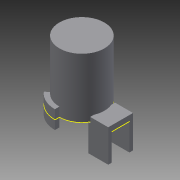
# Autodesk Inventor part: 知能ロボコンシリンダ延長
Saved by Autodesk Inventor 2013 (Build 170138000, 138)
## iProperties
Created: 2014-06-19
Part Number: 知能ロボコンシリンダ延長
Material: 一般
Document SubType Name: Modeling
Designer: horumo136
Density: 1 g/cm^3
Author: horumo136
Autodesk Inventor part; units mm, degrees
ref_plane "YZ Plane" through (0, 0, 0) normal (1, 0, 0) x (0, 1, 0)
ref_plane "XZ Plane" through (0, 0, 0) normal (0, 1, 0) x (-1, 0, 0)
ref_plane "XY Plane" through (0, 0, 0) normal (0, 0, 1) x (1, 0, 0)
sketch "スケッチ1" plane through (0, 0, 0) normal (1, 0, 0) x (0, 1, 0)
  line L0 (-4.884, 7.5) -> (4.884, 7.5)
  line L1 (4.884, 7.5) -> (4.884, -7.5)
  line L2 (4.884, -7.5) -> (-4.884, -7.5)
  line L3 (-4.884, -7.5) -> (-4.884, 7.5)
  line L4 (-4.884, 7.5) -> (4.884, -7.5) construction
  line L5 (4.884, 7.5) -> (-4.884, -7.5) construction
  line L6 (-4.884, -7.5) -> (-6.884, -7.5)
  line L7 (-6.884, -7.5) -> (-6.884, 10.5)
  line L8 (-6.884, 10.5) -> (6.884, 10.5)
  line L9 (6.884, 10.5) -> (6.884, -7.5)
  line L10 (6.884, -7.5) -> (4.884, -7.5)
  point P0 (0, 0)
  dimension "d0" = 9.768
  dimension "d1" = 15
  dimension "d2" = 2
  dimension "d3" = 18
  dimension "d4" = 13.768
  constraints: 22 end point, 4 parallel, 3 perpendicular, 2 midpoint, 1 collinear, 1 horizontal
  measures "d0" distance of L1.end L2.end
  measures "d1" distance of L0.end L1.end
  measures "d2" distance of L2.end L6.end
  measures "d3" distance of L6.end L7.end
  measures "d4" distance of L7.end L8.end
extrude "押し出し1" add sketch "スケッチ1" along normal blind 10 contours L3 L6 L7 L8 L9 L10 L1 L0
sketch "スケッチ2" plane through (0, -6.884, 10.5) normal (0, 0, 1) x (1, 0, 0)
  line L0 (0, 13.768) -> (0, 0) projected
  line L1 (0, 0) -> (0, 2)
  line L2 (0, 13.768) -> (0, 11.768)
  line L3 (0, 11.768) -> (-11.5063, 6.8839)
  line L4 (0, 11.768) -> (12.5, 11.768) construction
  line L5 (0, 2) -> (-11.5063, 6.8839)
  circle A0 centre (-11.5063, 6.8839) radius 12.4999
  point P0 (0, 6.884)
  dimension "d7" = 2
  dimension "d8" = 2
  dimension "d9" = 12.5
  dimension "d10" = 157
  constraints: 10 end point, 2 point on line, 1 coincident, 1 equal length, 1 horizontal, 3 other
  measures "d7" distance of L0.end L1.end
  measures "d8" distance of L0.start L2.end
  measures "d9" distance of L2.end L3.end
  measures "d10" angle of L3 L4
extrude "押し出し2" add sketch "スケッチ2" along normal blind 30
sketch "スケッチ3" plane through (0, -6.884, 10.5) normal (0, 0, -1) x (-1, 0, 0)
  line L0 (0, 11.7677) -> (0, 2) projected
  arc A0 (0, 2) -> (0, 11.7677) centre (11.5063, 6.8839) ccw projected
  point P0 (0, 6.884)
extrude "押し出し3" add sketch "スケッチ3" along normal blind 3
sketch "スケッチ4" plane through (10, 4.884, 7.5) normal (0, 0, -1) x (-1, 0, 0)
  arc A0 (10, -9.768) -> (10, -0.0003) centre (21.5063, -4.8841) ccw projected
  line L0 (21.5063, -4.8841) -> (27.7563, 5.9411)
  line L1 (21.5063, -4.8841) -> (34.0062, -4.8841) construction
  line L2 (21.5063, -4.8841) -> (27.7563, -15.7094)
  line L3 (21.5063, -4.8841) -> (21.5063, 7.6158)
  line L4 (21.5063, -4.8841) -> (34.0062, -4.8841) construction
  line L5 (21.5063, -4.8841) -> (21.5063, 10.1159)
  line L6 (21.5063, -4.8841) -> (32.997, 4.7577)
  line L7 (21.5063, -4.8841) -> (36.5063, -4.8841) construction
  arc A1 (32.997, 4.7577) -> (21.5063, 10.1159) centre (21.5063, -4.8841) ccw
  line L8 (21.5063, -4.8841) -> (21.5063, -19.8841)
  line L9 (21.5063, -4.8841) -> (32.997, -14.526)
  arc A2 (21.5063, -19.8841) -> (32.997, -14.526) centre (21.5063, -4.8841) ccw
  point P0 (10, -4.884)
  dimension "d15" = 60
  dimension "d16" = 90
  dimension "d18" = 15
  dimension "d19" = 40
  constraints: 20 end point, 7 point on circle, 3 equal length, 3 horizontal, 2 centre point, 2 coincident, 2 symmetric about line, 1 collinear, 1 other
  measures "d15" angle of L1 L0
  measures "d16" angle of L4 L3
  measures "d18" distance of L0.start L6.end
  measures "d19" angle of L7 L6
extrude "押し出し4" add sketch "スケッチ4" against normal blind 5 contours L0 L3 A0 | A0 L5 A1 L6 | A0 L6 L0 | L9 A0 L2 | L2 A0 L8 | L9 A2 L8 A0
sketch "スケッチ5" plane through (10, 4.884, 7.5) normal (0, 0, -1) x (-1, 0, 0)
  arc A0 (31.0818, -12.9189) -> (31.0818, 3.1506) centre (21.5063, -4.8841) ccw projected
  line L0 (31.0818, 3.1506) -> (32.997, 4.7577) projected
  arc A1 (32.997, 4.7577) -> (21.5063, 10.1159) centre (21.5063, -4.8841) ccw projected
  line L1 (21.5063, 10.1159) -> (21.5063, 7.6158) projected
  arc A2 (21.5063, 7.6158) -> (10, -0.0003) centre (21.5063, -4.8841) ccw projected
  line L2 (10, -0.0003) -> (10, 0) projected
  line L3 (10, 0) -> (0, 0) projected
  line L4 (0, -9.768) -> (0, 0) projected
  line L5 (10, -9.768) -> (0, -9.768) projected
  arc A3 (10, -9.768) -> (21.5063, -17.384) centre (21.5063, -4.8841) ccw projected
  line L6 (21.5063, -17.384) -> (21.5063, -19.8841) projected
  arc A4 (21.5063, -19.8841) -> (32.997, -14.526) centre (21.5063, -4.8841) ccw projected
  line L7 (32.997, -14.526) -> (31.0818, -12.9189) projected
  point P0 (10, -4.884)
sketch "スケッチ6" plane through (10, 4.884, 7.5) normal (0, 0, -1) x (-1, 0, 0)
  line L0 (31.0818, 3.1506) -> (32.997, 4.7577) projected
  line L1 (21.5063, 10.1159) -> (21.5063, 7.6158) projected
  line L2 (10, -0.0003) -> (10, 0) projected
  line L3 (21.5063, -17.384) -> (21.5063, -19.8841) projected
  arc A0 (21.5063, -19.8841) -> (32.997, -14.526) centre (21.5063, -4.8841) ccw projected
  line L4 (32.997, -14.526) -> (31.0818, -12.9189) projected
  line L5 (21.5063, 10.1159) -> (21.5063, 7.6158)
  line L6 (32.997, 4.7577) -> (31.0818, 3.1506)
  line L7 (31.0818, -12.9189) -> (32.997, -14.526)
  line L8 (21.5063, -17.384) -> (21.5063, -19.8841)
  arc A1 (32.997, 4.7577) -> (21.5063, 10.1159) centre (21.5063, -4.8841) ccw
  arc A2 (21.5063, -19.8841) -> (32.997, -14.526) centre (21.5063, -4.8841) ccw
  arc A3 (21.5063, -17.3841) -> (31.0819, -12.919) centre (21.5063, -4.8841) ccw
  arc A4 (31.0819, 3.1507) -> (21.5063, 7.6159) centre (21.5063, -4.8841) ccw
  point P0 (10, -4.884)
  constraints: 9 end point, 8 point on circle, 4 centre point, 4 collinear, 4 point on line, 1 coincident, 1 concentric
extrude "押し出し5" add sketch "スケッチ6" along normal blind 5
sketch "スケッチ7" plane through (10, 4.884, 7.5) normal (0, 0, -1) x (-1, 0, 0)
  arc A0 (21.5063, 7.6158) -> (10, -0.0003) centre (21.5063, -4.8841) ccw projected
  line L0 (10, -9.768) -> (0, -9.768) projected
  arc A1 (10, -9.768) -> (21.5063, -17.384) centre (21.5063, -4.8841) ccw projected
  line L1 (21.5063, -17.384) -> (21.5063, -17.3841) projected
  arc A2 (21.5063, -17.3841) -> (31.0819, -12.919) centre (21.5063, -4.8841) ccw projected
  line L2 (10, 0) -> (10, 2)
  line L3 (10, 2) -> (11.0729, 2)
  arc A3 (11.0729, 2) -> (10, 0) centre (21.5048, -4.884) ccw
  arc A4 (10, -9.7677) -> (10.0001, -9.768) centre (21.5063, -4.8839) ccw
  line L4 (10, -9.768) -> (10, -9.7683)
  line L5 (11.0727, -11.768) -> (11.0729, -11.768)
  line L6 (10.0001, -9.768) -> (10.0001, -11.768)
  line L7 (10.0001, -11.768) -> (11.0727, -11.768)
  arc A5 (10.0001, -9.768) -> (11.0727, -11.768) centre (21.4959, -4.8904) ccw
  point P0 (10, -4.884)
  dimension "d25" = 2
  constraints: 12 end point, 9 point on circle, 3 centre point, 2 parallel, 2 perpendicular, 1 point on line
  measures "d25" distance of L2.start L2.end
extrude "押し出し6" add sketch "スケッチ7" along normal blind 15 contours A0 L2 L3 | A1 L7 L6
